Autodesk Fusion 360 part; units mm, degrees
(part 2 of 5)
  line L99 (217.2044, 94.7987, -0.5425) -> (214.1574, 88.9606, -0.5425)
  line L100 (229.1883, 17.794, -0.5425) -> (214.0829, 45.1294, -0.5425)
  line L101 (210.1198, 46.3093, -0.5425) -> (201.6545, 41.8242, -0.5425)
  line L102 (293.4635, 57.0179, -0.5425) -> (293.4635, 72.1916, -0.5425)
  arc A98 through (216.7158, 52.5703, -0.5425) (214.8476, 50.3729, -0.5425) (215.1327, 47.5028, -0.5425)
  arc A99 through (214.1574, 88.9606, -0.5425) (214.0147, 86.5484, -0.5425) (215.7224, 84.8389, -0.5425)
  line L103 (226.5548, 84.1235, -0.5425) -> (230.7717, 91.8438, -0.5425)
  line L104 (201.0039, 43.5591, -0.5425) -> (211.2158, 49.0246, -0.5425)
  line L105 (199.3291, 37.4177, -0.5425) -> (201.7431, 16.0362, -0.5425)
  line L106 (208.6237, 83.9074, -0.5425) -> (198.0965, 82.5311, -0.5425)
  line L107 (231.3102, 98.4094, -0.5425) -> (230.7073, 100.1344, -0.5425)
  line L108 (222.0557, 80.2922, -0.5425) -> (213.4569, 83.3852, -0.5425)
  arc A100 through (296.5336, 106.6129, -0.5425) (295.8856, 108.1774, -0.5425) (294.3211, 108.8254, -0.5425)
  line L109 (215.1327, 47.5028, -0.5425) -> (232.5299, 15.7176, -0.5425)
  arc A101 through (273.8579, 106.3021, -0.5425) (270.4819, 104.7377, -0.5425) (269.4929, 101.1507, -0.5425)
  line L110 (235.2375, 65.7635, -0.5425) -> (228.2248, 77.4788, -0.5425)
  arc A102 through (211.2158, 49.0246, -0.5425) (213.0904, 51.5465, -0.5425) (212.3403, 54.5979, -0.5425)
  arc A103 through (292.1232, 53.2736, -0.5425) (293.1183, 55.0294, -0.5425) (293.4635, 57.0179, -0.5425)
  arc A104 through (196.4178, 13.4172, -0.5425) (198.5944, 14.376, -0.5425) (199.3562, 16.6291, -0.5425)
  arc A105 through (233.851, 97.2274, -0.5425) (234.7613, 95.834, -0.5425) (236.1917, 94.9829, -0.5425)
  line L111 (268.8676, 90.1351, -0.5425) -> (266.9865, 102.5405, -0.5425)
  line L112 (232.4628, 66.2602, -0.5425) -> (226.309, 76.7604, -0.5425)
  line L113 (274.4552, 82.2574, -0.5425) -> (287.9958, 78.9742, -0.5425)
  arc A106 through (235.8049, 106.3021, -0.5425) (232.7822, 104.7266, -0.5425) (232.3424, 101.3464, -0.5425)
  arc A107 through (231.2263, 62.1248, -0.5425) (232.744, 63.9235, -0.5425) (232.4628, 66.2602, -0.5425)
  arc A108 through (215.5, 95.6328, -0.5425) (215.8168, 97.3721, -0.5425) (215.0822, 98.9802, -0.5425)
  line L114 (211.2519, 87.5615, -0.5425) -> (215.5, 95.6328, -0.5425)
  arc A109 through (222.0059, 82.4452, -0.5425) (224.595, 82.4316, -0.5425) (226.5548, 84.1235, -0.5425)
  arc A110 through (209.3714, 105.3255, -0.5425) (208.3789, 106.0469, -0.5425) (207.1787, 106.3021, -0.5425)
  line L115 (232.339, 60.3964, -0.5425) -> (216.7158, 52.5703, -0.5425)
  line L116 (215.7224, 84.8389, -0.5425) -> (222.0059, 82.4452, -0.5425)
  arc A111 through (209.0833, 86.0187, -0.5425) (210.3515, 86.5316, -0.5425) (211.2519, 87.5615, -0.5425)
  arc A112 through (201.7431, 16.0362, -0.5425) (202.7091, 14.1673, -0.5425) (204.6745, 13.4172, -0.5425)
  spline S0 degree 5 poles (37.6621, 101.8013, -0.5425) (37.9412, 101.8066, -0.5298) (38.4481, 101.843, -0.5085) (39.0545, 101.9753, -0.4883) (39.5781, 102.2952, -0.4831) (39.8825, 102.8688, -0.5029) (39.9929, 103.5346, -0.5365) (40.0648, 104.211, -0.5713) (40.2254, 104.8318, -0.5972) (40.5423, 105.3622, -0.609) (41.0432, 105.7885, -0.6044) (41.5947, 106.045, -0.5876) (42.0909, 106.1912, -0.5678) (42.4578, 106.2685, -0.5514) (42.6502, 106.3021, -0.5425) knots 0 0 0 0 0 0 0.1 0.2 0.3 0.4 0.5 0.6 0.7 0.8 0.9 1 1 1 1 1 1
  line L117 (36.4174, 101.7778, -0.5988) -> (38.9069, 101.8248, -0.4861)
  line L118 (65.0016, 71.3547, -0.5425) -> (79.0443, 79.8182, -0.5425)
  point P0 (207.0175, 69.7948)
  point P1 (207.0175, 69.7948)
  point P2 (40.091, 104.2207)
ref_plane "WorkPlane3" through (-60.7921, 150, 14.512) normal (0.12473, 0, 0.992191) x (0, 1, 0)
sketch "Sketch13" plane through (0.8502, 0, 6.7629) normal (0.12473, 0, 0.992191) x (0, 1, 0)
  arc A0 through (128.5492, 107.9276, -0.5425) (126.6265, 107.2149, -0.5425) (125.6327, 105.4212, -0.5425)
  arc A1 through (146.4088, 56.3524, -0.5425) (149.6864, 55.4797, -0.5425) (152.619, 57.1839, -0.5425)
  arc A2 through (13.5344, 103.4268, -0.5425) (11.1356, 102.4332, -0.5425) (10.1419, 100.0343, -0.5425)
  line L0 (10.1419, 65.1989, -0.5425) -> (10.1419, 18.7302, -0.5425)
  arc A3 through (13.9723, 85.5184, -0.5425) (11.3447, 85.0798, -0.5425) (10.1419, 82.7029, -0.5425)
  arc A4 through (156.4587, 58.9806, -0.5425) (155.942, 56.5284, -0.5425) (157.4975, 54.5636, -0.5425)
  line L1 (294.3211, 12.6445, -0.5425) -> (9.3501, 12.6445, -0.5425)
  line L2 (10.1419, 100.0343, -0.5425) -> (10.1419, 91.4948, -0.5425)
  arc A5 through (123.35, 103.697, -0.5425) (122.4956, 106.6479, -0.5425) (119.7027, 107.9276, -0.5425)
  arc A6 through (10.1419, 18.7302, -0.5425) (11.222, 16.1227, -0.5425) (13.8294, 15.0427, -0.5425)
  arc A7 through (103.6411, 44.2546, -0.5425) (106.2902, 44.6336, -0.5425) (107.543, 46.9984, -0.5425)
  arc A8 through (116.5331, 76.1094, -0.5425) (112.392, 76.5395, -0.5425) (110.1305, 73.0437, -0.5425)
  arc A9 through (9.3501, 110.4509, -0.5425) (7.7856, 109.8029, -0.5425) (7.1376, 108.2384, -0.5425)
  line L3 (120.1949, 82.505, -0.5425) -> (123.35, 103.697, -0.5425)
  line L4 (125.6327, 105.4212, -0.5425) -> (121.5744, 78.7404, -0.5425)
  line L5 (10.9643, 77.8757, -0.5425) -> (50.5643, 16.3952, -0.5425)
  line L6 (108.7653, 39.733, -0.5425) -> (125.8648, 19.9201, -0.5425)
  line L7 (110.1305, 73.0437, -0.5425) -> (109.448, 44.8203, -0.5425)
  arc A10 through (115.2719, 78.7654, -0.5425) (118.4948, 79.6329, -0.5425) (120.1949, 82.505, -0.5425)
  line L8 (12.6248, 88.1163, -0.5425) -> (62.0516, 72.6514, -0.5425)
  line L9 (45.4146, 20.7352, -0.5425) -> (15.5677, 66.8029, -0.5425)
  line L10 (9.3501, 14.8498) -> (294.6499, 14.8498)
  line L11 (9.3501, 110.4509, -0.5425) -> (294.3211, 110.4509, -0.5425)
  arc A11 through (107.9965, 74.659, -0.5425) (107.159, 76.9469, -0.5425) (105.004, 78.0835, -0.5425)
  arc A12 through (121.5744, 78.7404, -0.5425) (121.89, 76.034, -0.5425) (123.5394, 73.8653, -0.5425)
  arc A13 through (15.5677, 66.8029, -0.5425) (12.2556, 68.0278, -0.5425) (10.1419, 65.1989, -0.5425)
  arc A14 through (127.0398, 21.5138, -0.5425) (129.4645, 20.4975, -0.5425) (131.7372, 21.8193, -0.5425)
  arc A15 through (109.448, 44.8203, -0.5425) (109.8778, 42.1553, -0.5425) (111.2377, 39.8234, -0.5425)
  line L12 (153.5813, 51.294, -0.5425) -> (133.0891, 19.5942, -0.5425)
  line L13 (61.4337, 70.6789, -0.5425) -> (13.9723, 85.5184, -0.5425)
  arc A16 through (108.7653, 39.733, -0.5425) (107.7529, 40.6338, -0.5425) (106.5409, 41.2402, -0.5425)
  line L14 (123.5394, 73.8653, -0.5425) -> (146.4088, 56.3524, -0.5425)
  line L15 (13.8294, 15.0427, -0.5425) -> (42.3199, 15.0427, -0.5425)
  line L16 (111.2377, 39.8234, -0.5425) -> (127.0398, 21.5138, -0.5425)
  line L17 (37.6621, 103.4268, -0.5425) -> (13.5344, 103.4268, -0.5425)
  arc A17 (7.1376, 17.0623) -> (9.3501, 14.8498) centre (9.3501, 17.0623) ccw
  arc A18 through (70.492, 52.7161, -0.5425) (70.5116, 54.0318, -0.5425) (70.1435, 55.2951, -0.5425)
  line L18 (131.7372, 21.8193, -0.5425) -> (148.5132, 47.3064, -0.5425)
  line L19 (172.3385, 107.9276, -0.5425) -> (128.5492, 107.9276, -0.5425)
  line L20 (156.4587, 58.9806, -0.5425) -> (176.5219, 85.5722, -0.5425)
  line L21 (296.8624, 17.0623) -> (296.8624, 110.4437)
  arc A19 through (180.1276, 15.0427, -0.5425) (182.5336, 16.2858, -0.5425) (182.9119, 18.9675, -0.5425)
  line L22 (236.4115, 15.0427, -0.5425) -> (249.3606, 15.0427, -0.5425)
  arc A20 through (214.0829, 46.7549, -0.5425) (212.3427, 48.1555, -0.5425) (210.1198, 47.9348, -0.5425)
  line L23 (236.9767, 94.2988, -0.5425) -> (263.2633, 85.8479, -0.5425)
  arc A21 through (239.2829, 63.0131, -0.5425) (235.7303, 63.0824, -0.5425) (232.339, 62.0219, -0.5425)
  arc A22 through (235.2375, 67.389, -0.5425) (236.4809, 66.0477, -0.5425) (238.1606, 65.3238, -0.5425)
  line L24 (201.0039, 45.1846, -0.5425) -> (211.2158, 50.6501, -0.5425)
  line L25 (204.6745, 15.0427, -0.5425) -> (226.6063, 15.0427, -0.5425)
  line L26 (191.3482, 44.4035, -0.5425) -> (178.6355, 45.2846, -0.5425)
  line L27 (262.6115, 107.9276, -0.5425) -> (235.8049, 107.9276, -0.5425)
  line L28 (249.4163, 63.057, -0.5425) -> (238.1606, 65.3238, -0.5425)
  arc A23 through (196.4178, 15.0427, -0.5425) (198.5944, 16.0015, -0.5425) (199.3562, 18.2546, -0.5425)
  line L29 (236.1917, 96.6084, -0.5425) -> (264.0999, 87.6951, -0.5425)
  arc A24 through (175.2679, 40.8003, -0.5425) (173.7034, 43.4764, -0.5425) (171.2495, 45.3704, -0.5425)
  line L30 (248.8594, 61.2625, -0.5425) -> (239.2829, 63.0131, -0.5425)
  arc A25 through (213.8317, 57.7017, -0.5425) (215.4931, 56.6815, -0.5425) (217.428, 56.9204, -0.5425)
  line L31 (210.1198, 47.9348, -0.5425) -> (201.6545, 43.4497, -0.5425)
  line L32 (256.3019, 30.8271, -0.5425) -> (252.4432, 57.5422, -0.5425)
  line L33 (229.1883, 19.4195, -0.5425) -> (214.0829, 46.7549, -0.5425)
  line L34 (190.7528, 73.975, -0.5425) -> (196.7325, 47.1438, -0.5425)
  line L35 (254.2531, 57.8338, -0.5425) -> (258.1218, 32.1079, -0.5425)
  line L36 (196.1913, 79.369, -0.5425) -> (213.8317, 57.7017, -0.5425)
  line L37 (212.3403, 56.2234, -0.5425) -> (195.9237, 76.4744, -0.5425)
  line L38 (275.8299, 35.0581, -0.5425) -> (292.1232, 54.8991, -0.5425)
  line L39 (296.5336, 108.2384, -0.5425) -> (296.5336, 14.857, -0.5425)
  line L40 (300.5325, 116.9713, -0.5425) -> (300.5325, 7.1103, -0.5425)
  line L41 (261.9665, 29.7462, -0.5425) -> (273.8014, 33.6658, -0.5425)
  arc A26 through (294.3211, 12.6445, -0.5425) (295.8856, 13.2925, -0.5425) (296.5336, 14.857, -0.5425)
  line L42 (274.4552, 83.8829, -0.5425) -> (287.9958, 80.5997, -0.5425)
  line L43 (289.9863, 78.1394, -0.5425) -> (277.0376, 80.9788, -0.5425)
  arc A27 through (293.4635, 47.0663, -0.5425) (291.9967, 49.1493, -0.5425) (289.5412, 48.4704, -0.5425)
  arc A28 through (290.5135, 15.0427, -0.5425) (292.5995, 15.9067, -0.5425) (293.4635, 17.9927, -0.5425)
  arc A29 through (176.2747, 88.2323, -0.5425) (177.0332, 89.7841, -0.5425) (177.1399, 91.508, -0.5425)
  line L44 (289.0385, 107.9276, -0.5425) -> (273.8579, 107.9276, -0.5425)
  line L45 (187.1226, 81.2581, -0.5425) -> (194.4335, 47.9794, -0.5425)
  arc A30 through (175.2618, 105.3735, -0.5425) (174.2794, 107.1991, -0.5425) (172.3385, 107.9276, -0.5425)
  line L46 (232.4628, 67.8857, -0.5425) -> (226.309, 78.3859, -0.5425)
  arc A31 through (180.3167, 107.9276, -0.5425) (178.0915, 106.9144, -0.5425) (177.3948, 104.5708, -0.5425)
  line L47 (255.7129, 18.0094, -0.5425) -> (257.7618, 23.6594, -0.5425)
  arc A32 through (79.0291, 81.4345, -0.5425) (80.4163, 82.7098, -0.5425) (81.1941, 84.4262, -0.5425)
  arc A33 through (85.3097, 80.4194, -0.5425) (82.1977, 80.2707, -0.5425) (79.3035, 79.1172, -0.5425)
  arc A34 through (67.2556, 20.1909, -0.5425) (68.2461, 16.6058, -0.5425) (71.6211, 15.0427, -0.5425)
  arc A35 through (64.1302, 68.3113, -0.5425) (63.0327, 69.7807, -0.5425) (61.4337, 70.6789, -0.5425)
  arc A36 (294.6499, 14.8498) -> (296.8624, 17.0623) centre (294.6499, 17.0623) ccw
  line L48 (77.6309, 51.2153, -0.5425) -> (106.5409, 41.2402, -0.5425)
  line L49 (85.3097, 80.4194, -0.5425) -> (105.004, 78.0835, -0.5425)
  line L50 (119.7027, 107.9276, -0.5425) -> (92.2179, 107.9276, -0.5425)
  line L51 (103.6411, 44.2546, -0.5425) -> (75.7593, 53.7636, -0.5425)
  line L52 (87.1104, 82.2687, -0.5425) -> (115.2719, 78.7654, -0.5425)
  line L53 (123.6315, 15.0427, -0.5425) -> (71.6211, 15.0427, -0.5425)
  arc A37 through (157.3818, 52.3291, -0.5425) (155.2835, 52.5387, -0.5425) (153.5813, 51.294, -0.5425)
  line L54 (3.4675, 116.9713, -0.5425) -> (300.5325, 116.9713, -0.5425)
  arc A38 through (216.7158, 54.1958, -0.5425) (214.8476, 51.9984, -0.5425) (215.1327, 49.1283, -0.5425)
  arc A39 through (196.7325, 47.1438, -0.5425) (198.3819, 45.1041, -0.5425) (201.0039, 45.1846, -0.5425)
  line L55 (173.0748, 46.7985, -0.5425) -> (157.4975, 54.5636, -0.5425)
  arc A40 through (181.0984, 42.9156, -0.5425) (178.5412, 41.7629, -0.5425) (178.1042, 38.9921, -0.5425)
  arc A41 through (173.0748, 46.7985, -0.5425) (175.7805, 45.7673, -0.5425) (178.6355, 45.2846, -0.5425)
  line L56 (135.5665, 15.0427, -0.5425) -> (180.1276, 15.0427, -0.5425)
  line L57 (178.1042, 38.9921, -0.5425) -> (185.8555, 17.0116, -0.5425)
  line L58 (217.428, 56.9204, -0.5425) -> (231.2263, 63.7503, -0.5425)
  line L59 (232.339, 62.0219, -0.5425) -> (216.7158, 54.1958, -0.5425)
  arc A42 through (201.6545, 43.4497, -0.5425) (199.8127, 41.6049, -0.5425) (199.3291, 39.0432, -0.5425)
  arc A43 through (61.1239, 15.0427, -0.5425) (63.5088, 15.9177, -0.5425) (64.7618, 18.1275, -0.5425)
  arc A44 through (50.5643, 16.3952, -0.5425) (51.6319, 15.4028, -0.5425) (53.0443, 15.0427, -0.5425)
  arc A45 through (77.6309, 51.2153, -0.5425) (73.9232, 50.8341, -0.5425) (71.8221, 47.7555, -0.5425)
  line L60 (64.7618, 18.1275, -0.5425) -> (70.492, 52.7161, -0.5425)
  line L61 (53.0443, 15.0427, -0.5425) -> (61.1239, 15.0427, -0.5425)
  line L62 (88.0477, 104.6024, -0.5425) -> (83.9707, 86.7489, -0.5425)
  line L63 (71.4916, 57.5515, -0.5425) -> (66.9703, 66.9675, -0.5425)
  line L64 (81.7514, 107.9276, -0.5425) -> (42.6502, 107.9276, -0.5425)
  arc A46 through (68.665, 72.6667, -0.5425) (66.7178, 70.1441, -0.5425) (66.9703, 66.9675, -0.5425)
  arc A47 through (71.4916, 57.5515, -0.5425) (73.2442, 55.228, -0.5425) (75.7593, 53.7636, -0.5425)
  arc A48 through (232.5299, 17.3431, -0.5425) (234.1555, 15.661, -0.5425) (236.4115, 15.0427, -0.5425)
  arc A49 through (201.7431, 17.6617, -0.5425) (202.7091, 15.7928, -0.5425) (204.6745, 15.0427, -0.5425)
  arc A50 through (231.2263, 63.7503, -0.5425) (232.744, 65.549, -0.5425) (232.4628, 67.8857, -0.5425)
  line L65 (199.3291, 39.0432, -0.5425) -> (201.7431, 17.6617, -0.5425)
  line L66 (199.3562, 18.2546, -0.5425) -> (197.4845, 39.2503, -0.5425)
  arc A51 through (211.2158, 50.6501, -0.5425) (213.0904, 53.172, -0.5425) (212.3403, 56.2234, -0.5425)
  line L67 (171.2495, 45.3704, -0.5425) -> (157.3818, 52.3291, -0.5425)
  line L68 (7.1376, 110.4437) -> (7.1376, 17.0623)
  arc A52 through (62.0516, 72.6514, -0.5425) (63.5927, 72.5096, -0.5425) (65.0563, 73.0125, -0.5425)
  arc A53 through (42.3199, 15.0427, -0.5425) (45.5596, 16.9689, -0.5425) (45.4146, 20.7352, -0.5425)
  line L69 (81.1941, 84.4262, -0.5425) -> (85.4902, 103.2388, -0.5425)
  line L70 (68.665, 72.6667, -0.5425) -> (79.3035, 79.1172, -0.5425)
  arc A54 through (83.9707, 86.7489, -0.5425) (84.5459, 83.8117, -0.5425) (87.1104, 82.2687, -0.5425)
  line L71 (67.2556, 20.1909, -0.5425) -> (71.8221, 47.7555, -0.5425)
  line L72 (65.0016, 72.9802, -0.5425) -> (79.0443, 81.4437, -0.5425)
  line L73 (70.1435, 55.2951, -0.5425) -> (64.1302, 68.3113, -0.5425)
  arc A55 through (85.4902, 103.2388, -0.5425) (84.7499, 106.4835, -0.5425) (81.7514, 107.9276, -0.5425)
  arc A56 through (92.2179, 107.9276, -0.5425) (89.5511, 106.9945, -0.5425) (88.0477, 104.6024, -0.5425)
  arc A57 through (226.6063, 15.0427, -0.5425) (229.1471, 16.4937, -0.5425) (229.1883, 19.4195, -0.5425)
  arc A58 through (191.3482, 44.4035, -0.5425) (193.7858, 45.4194, -0.5425) (194.4335, 47.9794, -0.5425)
  arc A59 through (197.4845, 39.2503, -0.5425) (196.6144, 41.092, -0.5425) (194.7583, 41.9308, -0.5425)
  line L74 (215.1327, 49.1283, -0.5425) -> (232.5299, 17.3431, -0.5425)
  line L75 (194.7583, 41.9308, -0.5425) -> (181.0984, 42.9156, -0.5425)
  arc A60 through (185.8555, 17.0116, -0.5425) (186.9334, 15.5847, -0.5425) (188.6375, 15.0427, -0.5425)
  arc A61 through (133.0891, 19.5942, -0.5425) (132.9755, 16.5823, -0.5425) (135.5665, 15.0427, -0.5425)
  line L76 (276.3301, 32.1764, -0.5425) -> (290.2479, 30.3805, -0.5425)
  arc A62 through (276.3301, 32.1764, -0.5425) (275.6694, 32.187, -0.5425) (275.0229, 32.0503, -0.5425)
  line L77 (289.5412, 48.4704, -0.5425) -> (280.1951, 37.0893, -0.5425)
  arc A63 through (198.0965, 84.1566, -0.5425) (195.738, 82.3223, -0.5425) (196.1913, 79.369, -0.5425)
  arc A64 through (287.9958, 80.5997, -0.5425) (291.7741, 81.422, -0.5425) (293.4635, 84.9001, -0.5425)
  line L78 (261.9099, 27.6959, -0.5425) -> (275.0229, 32.0503, -0.5425)
  arc A65 through (293.4635, 26.7234, -0.5425) (292.5453, 29.1583, -0.5425) (290.2479, 30.3805, -0.5425)
  line L79 (180.9121, 89.4237, -0.5425) -> (188.1391, 86.2233, -0.5425)
  arc A66 through (265.809, 82.6487, -0.5425) (265.0201, 84.6334, -0.5425) (263.2633, 85.8479, -0.5425)
  line L80 (235.2375, 67.389, -0.5425) -> (228.2248, 79.1043, -0.5425)
  arc A67 through (280.1951, 37.0893, -0.5425) (279.848, 34.8702, -0.5425) (281.6207, 33.491, -0.5425)
  line L81 (182.035, 86.864, -0.5425) -> (183.2206, 86.2706, -0.5425)
  arc A68 through (290.9668, 32.2801, -0.5425) (292.7116, 32.8124, -0.5425) (293.4635, 34.4743, -0.5425)
  arc A69 through (255.7129, 18.0094, -0.5425) (255.9812, 15.9851, -0.5425) (257.7929, 15.0427, -0.5425)
  line L82 (253.5627, 18.0811, -0.5425) -> (255.7697, 24.7696, -0.5425)
  line L83 (208.6237, 85.5329, -0.5425) -> (198.0965, 84.1566, -0.5425)
  arc A70 through (209.3714, 106.951, -0.5425) (208.3789, 107.6724, -0.5425) (207.1787, 107.9276, -0.5425)
  arc A71 through (249.3606, 15.0427, -0.5425) (251.9533, 15.8818, -0.5425) (253.5627, 18.0811, -0.5425)
  line L84 (281.6207, 33.491, -0.5425) -> (290.9668, 32.2801, -0.5425)
  arc A72 through (292.1232, 54.8991, -0.5425) (293.1183, 56.6549, -0.5425) (293.4635, 58.6434, -0.5425)
  line L85 (293.4635, 34.4743, -0.5425) -> (293.4635, 47.0663, -0.5425)
  arc A73 through (255.7697, 24.7696, -0.5425) (256.3873, 27.7675, -0.5425) (256.3019, 30.8271, -0.5425)
  arc A74 through (258.1218, 32.1079, -0.5425) (259.4949, 30.033, -0.5425) (261.9665, 29.7462, -0.5425)
  line L86 (265.809, 82.6487, -0.5425) -> (265.9528, 80.9526, -0.5425)
  arc A75 through (273.8014, 33.6658, -0.5425) (274.9144, 34.2181, -0.5425) (275.8299, 35.0581, -0.5425)
  line L87 (264.5468, 76.607, -0.5425) -> (254.3494, 64.7515, -0.5425)
  arc A76 through (213.4569, 85.0107, -0.5425) (211.0714, 85.5603, -0.5425) (208.6237, 85.5329, -0.5425)
  arc A77 through (261.9099, 27.6959, -0.5425) (259.3727, 26.1536, -0.5425) (257.7618, 23.6594, -0.5425)
  line L88 (293.4635, 26.7234, -0.5425) -> (293.4635, 17.9927, -0.5425)
  arc A78 through (209.0833, 87.6442, -0.5425) (210.3515, 88.1571, -0.5425) (211.2519, 89.187, -0.5425)
  line L89 (290.5135, 15.0427, -0.5425) -> (257.7929, 15.0427, -0.5425)
  arc A79 through (249.4163, 63.057, -0.5425) (252.1126, 63.2354, -0.5425) (254.3494, 64.7515, -0.5425)
  line L90 (177.3948, 104.5708, -0.5425) -> (179.1848, 91.7143, -0.5425)
  line L91 (269.2803, 78.4929, -0.5425) -> (256.0736, 63.8745, -0.5425)
  arc A80 through (182.035, 86.864, -0.5425) (179.0447, 87.2154, -0.5425) (176.5219, 85.5722, -0.5425)
  arc A81 through (188.1391, 86.2233, -0.5425) (191.1487, 85.3739, -0.5425) (194.2757, 85.4006, -0.5425)
  line L92 (269.4929, 102.7762, -0.5425) -> (272.2404, 86.2656, -0.5425)
  line L93 (228.1101, 84.2056, -0.5425) -> (232.6022, 92.5381, -0.5425)
  arc A82 through (187.1226, 81.2581, -0.5425) (185.7389, 84.206, -0.5425) (183.2206, 86.2706, -0.5425)
  arc A83 through (179.1848, 91.7143, -0.5425) (179.7513, 90.3449, -0.5425) (180.9121, 89.4237, -0.5425)
  line L94 (207.1787, 107.9276, -0.5425) -> (180.3167, 107.9276, -0.5425)
  arc A84 through (220.6389, 100.0016, -0.5425) (218.6659, 98.4584, -0.5425) (217.2044, 96.4242, -0.5425)
  line L95 (194.2757, 85.4006, -0.5425) -> (209.0833, 87.6442, -0.5425)
  line L96 (177.1399, 91.508, -0.5425) -> (175.2618, 105.3735, -0.5425)
  line L97 (293.4635, 84.9001, -0.5425) -> (293.4635, 103.5026, -0.5425)
  arc A85 through (252.4432, 57.5422, -0.5425) (251.2505, 59.9796, -0.5425) (248.8594, 61.2625, -0.5425)
  arc A86 through (272.2404, 86.2656, -0.5425) (272.9897, 84.7413, -0.5425) (274.4552, 83.8829, -0.5425)
  arc A87 through (195.9237, 76.4744, -0.5425) (192.3483, 77.2728, -0.5425) (190.7528, 73.975, -0.5425)
  arc A88 through (236.9767, 94.2988, -0.5425) (234.4712, 94.2091, -0.5425) (232.6022, 92.5381, -0.5425)
  line L98 (226.5548, 85.749, -0.5425) -> (230.7717, 93.4693, -0.5425)
  line L99 (293.4635, 58.6434, -0.5425) -> (293.4635, 73.8171, -0.5425)
  line L100 (211.2519, 89.187, -0.5425) -> (215.5, 97.2583, -0.5425)
  line L101 (215.7224, 86.4644, -0.5425) -> (222.0059, 84.0707, -0.5425)
  arc A89 through (293.4635, 103.5026, -0.5425) (292.1675, 106.6315, -0.5425) (289.0385, 107.9276, -0.5425)
  arc A90 through (277.0376, 80.9788, -0.5425) (272.8243, 80.7801, -0.5425) (269.2803, 78.4929, -0.5425)
  arc A91 through (230.7073, 101.7599, -0.5425) (228.9517, 103.5512, -0.5425) (226.4521, 103.3439, -0.5425)
  arc A92 through (273.8579, 107.9276, -0.5425) (270.4819, 106.3632, -0.5425) (269.4929, 102.7762, -0.5425)
  arc A93 through (214.1574, 90.5861, -0.5425) (214.0147, 88.1739, -0.5425) (215.7224, 86.4644, -0.5425)
  arc A94 through (293.4635, 73.8171, -0.5425) (292.4863, 76.5907, -0.5425) (289.9863, 78.1394, -0.5425)
  arc A95 through (215.5, 97.2583, -0.5425) (215.8168, 98.9976, -0.5425) (215.0822, 100.6057, -0.5425)
  arc A96 through (296.5336, 108.2384, -0.5425) (295.8856, 109.8029, -0.5425) (294.3211, 110.4509, -0.5425)
  arc A97 through (222.0059, 84.0707, -0.5425) (224.595, 84.0571, -0.5425) (226.5548, 85.749, -0.5425)
  line L102 (232.3424, 102.9719, -0.5425) -> (233.851, 98.8529, -0.5425)
  line L103 (222.0557, 81.9177, -0.5425) -> (213.4569, 85.0107, -0.5425)
  arc A98 through (235.8049, 107.9276, -0.5425) (232.7822, 106.3521, -0.5425) (232.3424, 102.9719, -0.5425)
  line L104 (231.3102, 100.0349, -0.5425) -> (230.7073, 101.7599, -0.5425)
  arc A99 (296.8624, 110.4437) -> (294.6499, 112.6562) centre (294.6499, 110.4437) ccw
  arc A100 through (230.7717, 93.4693, -0.5425) (231.7374, 96.695, -0.5425) (231.3102, 100.0349, -0.5425)
  line L105 (217.2044, 96.4242, -0.5425) -> (214.1574, 90.5861, -0.5425)
  arc A101 through (226.309, 78.3859, -0.5425) (224.4925, 80.5253, -0.5425) (222.0557, 81.9177, -0.5425)
  line L106 (215.0822, 100.6057, -0.5425) -> (209.3714, 106.951, -0.5425)
  line L107 (268.8676, 91.7606, -0.5425) -> (266.9865, 104.166, -0.5425)
  arc A102 through (233.851, 98.8529, -0.5425) (234.7613, 97.4595, -0.5425) (236.1917, 96.6084, -0.5425)
  line L108 (226.4521, 103.3439, -0.5425) -> (220.6389, 100.0016, -0.5425)
  arc A103 through (256.0736, 63.8745, -0.5425) (254.4848, 61.0587, -0.5425) (254.2531, 57.8338, -0.5425)
  arc A104 through (264.5468, 76.607, -0.5425) (265.6874, 78.6383, -0.5425) (265.9528, 80.9526, -0.5425)
  arc A105 through (266.9865, 104.166, -0.5425) (265.4964, 106.8579, -0.5425) (262.6115, 107.9276, -0.5425)
  arc A106 through (264.0999, 87.6951, -0.5425) (267.6144, 88.4019, -0.5425) (268.8676, 91.7606, -0.5425)
  arc A107 through (228.1101, 84.2056, -0.5425) (227.4932, 81.6398, -0.5425) (228.2248, 79.1043, -0.5425)
  line L109 (182.9119, 18.9675, -0.5425) -> (175.2679, 40.8003, -0.5425)
  line L110 (188.6375, 15.0427, -0.5425) -> (196.4178, 15.0427, -0.5425)
  line L111 (152.619, 57.1839, -0.5425) -> (176.2747, 88.2323, -0.5425)
  line L112 (10.1419, 82.7029, -0.5425) -> (10.1419, 80.6712, -0.5425)
  line L113 (3.4675, 7.1103, -0.5425) -> (3.4675, 116.9713, -0.5425)
  arc A108 through (123.6315, 15.0427, -0.5425) (126.3137, 16.7645, -0.5425) (125.8648, 19.9201, -0.5425)
  arc A109 through (10.1419, 91.4948, -0.5425) (10.8294, 89.3984, -0.5425) (12.6248, 88.1163, -0.5425)
  line L114 (107.9965, 74.659, -0.5425) -> (107.543, 46.9984, -0.5425)
  arc A110 through (148.5132, 47.3064, -0.5425) (149.0689, 49.9488, -0.5425) (147.6751, 52.2615, -0.5425)
  arc A111 through (10.1419, 80.6712, -0.5425) (10.3518, 79.2143, -0.5425) (10.9643, 77.8757, -0.5425)
  line L115 (7.1376, 14.857, -0.5425) -> (7.1376, 108.2384, -0.5425)
  arc A112 through (7.1376, 14.857, -0.5425) (7.7856, 13.2925, -0.5425) (9.3501, 12.6445, -0.5425)
  line L116 (147.6751, 52.2615, -0.5425) -> (116.5331, 76.1094, -0.5425)
  line L117 (37.6527, 103.4268, -0.5425) -> (42.657, 107.9276, -0.5425)
  point P0 (207.0175, 71.4203)
  point P1 (207.0175, 71.4203)
extrude "Extrude4" cut sketch "Sketch13" against normal through all contours A0 A1 L4 A12 L14 L19 A29 A30 L96 L111 | A2 L2 L8 L17 A32 L64 A52 L69 L72 A55 A109 L117 | L0 A6 L9 A13 L15 A53 | A3 L5 L13 A18 A35 A43 A44 L60 L61 L73 L112 A111 | A4 L20 L26 L45 L55 A41 A58 L81 A80 A82 | A5 L3 A10 L50 L52 L62 A54 A56 | A7 A11 A33 L49 L51 L63 A46 A47 L70 L114 | A8 L7 A14 A15 L16 L18 A110 L116 | L6 A16 A34 L48 L53 A45 L71 A108 | L12 A19 A24 A37 L56 L67 A61 L109 | L22 A21 L30 L32 A38 L59 A48 L74 L82 A71 A73 A85 | A20 L25 L31 L33 A42 A49 L65 A57 | L23 A22 L28 A66 L80 L86 L87 A79 L93 A88 A104 A107 | L24 L34 L37 A39 A51 A87 | L27 L29 L102 A98 L107 A102 A105 A106 | A23 A40 L57 L66 A59 L75 A60 L110 | A25 L36 L46 L58 A50 A63 L83 A76 L103 A101 | L35 L38 L41 L43 A72 A74 A75 L91 L99 A90 A94 A103 | L42 L44 A64 L92 L97 A86 A89 A92 | A27 L77 A67 A68 L84 L85 | A28 L47 L76 A62 L78 A65 A69 A77 L88 L89 | A31 L79 A70 A78 L90 A81 A83 L94 L95 L100 A95 L106 | A84 L98 L101 A91 A93 A97 L104 A100 L105 L108 in plane through (0.7825, 0, 6.2246) normal (0.12473, 0, 0.992191)
sketch "Sketch14" plane through (0, 0, 0) normal (0, -1, 0) x (1, 0, 0)
  line L0 (-113.7873, 37.3) -> (-113.7873, 4.9975)
  line L1 (-113.7873, 4.9975) -> (-4.7873, 4.9975)
  line L2 (-4.7873, 4.9975) -> (-4.7873, 23.5975)
  line L3 (-4.7873, 23.5975) -> (-113.7873, 37.3)
sketch "Sketch15" plane through (0, 0, 0) normal (0, 0, 1) x (1, 0, 0)
  line L0 (5.3988, -2.1298) -> (5.3988, 1.5536)
  line L1 (5.3988, 1.5536) -> (6.4633, 1.4209)
  line L2 (6.4633, 1.4209) -> (6.0119, -2.2014)
  line L3 (6.0119, -2.2014) -> (5.3988, -2.1298)
  line L4 (5.4744, 1.348) -> (5.5749, 1.5095) construction
  line L5 (5.5749, 1.5095) -> (5.9354, 1.3104) construction
  line L6 (5.9354, 1.3104) -> (5.4453, 1.1367) construction
  line L7 (5.4453, 1.1367) -> (5.4378, 1.2494) construction
  line L8 (5.4378, 1.2494) -> (5.4744, 1.348) construction
  spline S0 degree 5 poles (5.4744, 1.348) (5.5749, 1.5095) (5.9354, 1.3104) (5.4453, 1.1367) (5.4378, 1.2494) (5.4744, 1.348) knots 0 0 0 0 0 0 1 1 1 1 1 1
  line L9 (6.0311, 1.103) -> (6.0048, 1.3059) construction
  line L10 (6.0048, 1.3059) -> (6.0442, 1.46) construction
  line L11 (6.0442, 1.46) -> (5.4771, 1.1925) construction
  line L12 (5.4771, 1.1925) -> (5.3709, 1.0098) construction
  line L13 (5.3709, 1.0098) -> (5.5225, 0.9394) construction
  line L14 (5.5225, 0.9394) -> (5.6861, 0.8534) construction
  line L15 (5.6861, 0.8534) -> (6.0526, 0.9979) construction
  line L16 (6.0526, 0.9979) -> (6.0311, 1.103) construction
  spline S1 degree 5 poles (6.0311, 1.103) (6.0048, 1.3059) (6.0442, 1.46) (5.4771, 1.1925) (5.3709, 1.0098) (5.5225, 0.9394) (5.6861, 0.8534) (6.0526, 0.9979) (6.0311, 1.103) knots 0 0 0 0 0 0 0.25 0.5 0.75 1 1 1 1 1 1
  line L17 (6.1058, 0.8886) -> (6.162, 0.6486)
  line L18 (6.2944, 0.6369) -> (6.2967, 0.642)
  line L19 (6.3105, 0.694) -> (6.3258, 0.826)
  line L20 (6.2336, 0.9612) -> (6.1918, 0.9722)
  arc A0 (6.1918, 0.9722) -> (6.1058, 0.8886) centre (6.1739, 0.9046) ccw
  arc A1 (6.162, 0.6486) -> (6.2944, 0.6369) centre (6.2301, 0.6646) ccw
  arc A2 (6.2967, 0.642) -> (6.3105, 0.694) centre (6.1268, 0.7153) ccw
  arc A3 (6.3258, 0.826) -> (6.2336, 0.9612) centre (6.2016, 0.8403) ccw
  line L21 (5.9923, 0.0338) -> (6.0698, -0.2718)
  line L22 (6.1873, -0.266) -> (6.2399, 0.0832)
  line L23 (6.2112, 0.22) -> (6.1931, 0.2485)
  line L24 (6.0168, 0.2345) -> (6.0062, 0.21)
  arc A4 (6.1931, 0.2485) -> (6.0168, 0.2345) centre (6.1086, 0.195) ccw
  arc A5 (6.0062, 0.21) -> (5.9923, 0.0338) centre (6.2588, 0.1014) ccw
  arc A6 (6.2399, 0.0832) -> (6.2112, 0.22) centre (6.0422, 0.1131) ccw
  arc A7 (6.0698, -0.2718) -> (6.1873, -0.266) centre (6.1279, -0.257) ccw
  line L25 (5.9776, -1.9957) -> (6.0438, -1.4551)
  line L26 (5.933, -1.3436) -> (5.8966, -1.3479)
  line L27 (5.6749, -1.4635) -> (5.5171, -1.6418)
  line L28 (5.4543, -1.8075) -> (5.4543, -1.9385)
  line L29 (5.5405, -2.0375) -> (5.8646, -2.0826)
  arc A8 (6.0438, -1.4551) -> (5.933, -1.3436) centre (5.9445, -1.443) ccw
  arc A9 (5.8966, -1.3479) -> (5.6749, -1.4635) centre (5.937, -1.6955) ccw
  arc A10 (5.5171, -1.6418) -> (5.4543, -1.8075) centre (5.7043, -1.8075) ccw
  arc A11 (5.8646, -2.0826) -> (5.9776, -1.9957) centre (5.8784, -1.9835) ccw
  arc A12 (5.4543, -1.9385) -> (5.5405, -2.0375) centre (5.5543, -1.9385) ccw
  line L30 (5.716, -0.8769) -> (5.7261, -1.2218)
  line L31 (5.6538, -1.4051) -> (5.5473, -1.5125)
  line L32 (5.4703, -1.4808) -> (5.4703, -0.8771)
  line L33 (5.5453, -0.7803) -> (5.5472, -0.7798)
  line L34 (5.5472, -0.7798) -> (5.6172, -0.7798)
  line L35 (5.6172, -0.7798) -> (5.6161, -0.7798)
  arc A13 (5.5453, -0.7803) -> (5.4703, -0.8771) centre (5.5703, -0.8771) ccw
  arc A14 (5.716, -0.8769) -> (5.6161, -0.7798) centre (5.6161, -0.8798) ccw
  arc A15 (5.6538, -1.4051) -> (5.7261, -1.2218) centre (5.4762, -1.2291) ccw
  arc A16 (5.4703, -1.4808) -> (5.5473, -1.5125) centre (5.5153, -1.4808) ccw
  line L36 (5.7779, -0.6031) -> (5.7773, -1.1532)
  line L37 (5.9091, -1.2844) -> (6.0011, -1.2758)
  line L38 (6.0011, -1.2758) -> (5.978, -1.278)
  line L39 (6.0677, -1.1924) -> (6.1601, -0.5408)
  line L40 (6.0692, -0.4571) -> (5.8557, -0.5057)
  arc A17 (5.7773, -1.1532) -> (5.8256, -1.2636) centre (5.9273, -1.1534) ccw
  arc A18 (5.8256, -1.2636) -> (5.9091, -1.2844) centre (5.897, -1.155) ccw
  arc A19 (5.8557, -0.5057) -> (5.7779, -0.6031) centre (5.8779, -0.6032) ccw
  arc A20 (5.978, -1.278) -> (6.0677, -1.1924) centre (5.9686, -1.1784) ccw
  arc A21 (6.1601, -0.5408) -> (6.0692, -0.4571) centre (6.0858, -0.5303) ccw
  line L41 (5.4668, -0.5654) -> (5.5025, -0.4813) construction
  line L42 (5.5025, -0.4813) -> (5.6981, -0.5066) construction
  line L43 (5.6981, -0.5066) -> (5.7507, -0.5528) construction
  line L44 (5.7507, -0.5528) -> (5.839, -0.8009) construction
  line L45 (5.839, -0.8009) -> (5.4416, -0.7358) construction
  line L46 (5.4416, -0.7358) -> (5.4668, -0.5654) construction
  spline S2 degree 5 poles (5.4668, -0.5654) (5.5025, -0.4813) (5.6981, -0.5066) (5.7507, -0.5528) (5.839, -0.8009) (5.4416, -0.7358) (5.4668, -0.5654) knots 0 0 0 0 0 0 0.5 1 1 1 1 1 1
  line L47 (5.4584, 0.0475) -> (5.4584, -0.329)
  line L48 (5.5834, -0.454) -> (5.6398, -0.454)
  line L49 (5.8754, -0.4279) -> (5.9471, -0.4118)
  line L50 (6.0217, -0.2878) -> (5.9448, -0.0066)
  line L51 (5.8693, 0.1148) -> (5.7172, 0.2492)
  line L52 (5.5703, 0.2333) -> (5.4776, 0.1064)
  arc A22 (5.4776, 0.1064) -> (5.4584, 0.0475) centre (5.5584, 0.0475) ccw
  arc A23 (5.7172, 0.2492) -> (5.5703, 0.2333) centre (5.651, 0.1743) ccw
  arc A24 (5.9448, -0.0066) -> (5.8693, 0.1148) centre (5.7037, -0.0725) ccw
  arc A25 (5.9471, -0.4118) -> (6.0217, -0.2878) centre (5.9252, -0.3142) ccw
  arc A26 (5.6398, -0.454) -> (5.8754, -0.4279) centre (5.6398, 0.621) ccw
  arc A27 (5.4584, -0.329) -> (5.5834, -0.454) centre (5.5834, -0.329) ccw
  line L53 (5.4649, 0.3902) -> (5.4649, 0.2831) construction
  line L54 (5.4649, 0.2831) -> (5.471, 0.2306) construction
  line L55 (5.471, 0.2306) -> (5.5942, 0.2286) construction
  line L56 (5.5942, 0.2286) -> (5.6366, 0.3538) construction
  line L57 (5.6366, 0.3538) -> (5.5518, 0.467) construction
  line L58 (5.5518, 0.467) -> (5.4649, 0.3902) construction
  spline S3 degree 5 poles (5.4649, 0.3902) (5.4649, 0.2831) (5.471, 0.2306) (5.5942, 0.2286) (5.6366, 0.3538) (5.5518, 0.467) (5.4649, 0.3902) knots 0 0 0 0 0 0 0.5 1 1 1 1 1 1
  line L59 (6.0183, 0.4104) -> (6.0284, 0.4589) construction
  line L60 (6.0284, 0.4589) -> (6.0769, 0.5134) construction
  line L61 (6.0769, 0.5134) -> (6.1557, 0.5033) construction
  line L62 (6.1557, 0.5033) -> (6.2001, 0.4286) construction
  line L63 (6.2001, 0.4286) -> (6.1436, 0.3458) construction
  line L64 (6.1436, 0.3458) -> (6.0345, 0.3498) construction
  line L65 (6.0345, 0.3498) -> (6.0183, 0.4104) construction
  spline S4 degree 5 poles (6.0183, 0.4104) (6.0284, 0.4589) (6.0769, 0.5134) (6.1557, 0.5033) (6.2001, 0.4286) (6.1436, 0.3458) (6.0345, 0.3498) (6.0183, 0.4104) knots 0 0 0 0 0 0 0.333333 0.666667 1 1 1 1 1 1
  line L66 (5.8042, 0.2629) -> (5.883, 0.1599) construction
  line L67 (5.883, 0.1599) -> (5.9598, 0.164) construction
  line L68 (5.9598, 0.164) -> (5.9961, 0.2932) construction
  line L69 (5.9961, 0.2932) -> (5.9699, 0.4245) construction
  line L70 (5.9699, 0.4245) -> (5.8406, 0.5659) construction
  line L71 (5.8406, 0.5659) -> (5.7517, 0.4972) construction
  line L72 (5.7517, 0.4972) -> (5.7133, 0.4003) construction
  line L73 (5.7133, 0.4003) -> (5.7214, 0.3114) construction
  line L74 (5.7214, 0.3114) -> (5.8042, 0.2629) construction
  spline S5 degree 5 poles (5.8042, 0.2629) (5.883, 0.1599) (5.9598, 0.164) (5.9961, 0.2932) (5.9699, 0.4245) (5.8406, 0.5659) (5.7517, 0.4972) (5.7133, 0.4003) (5.7214, 0.3114) (5.8042, 0.2629) knots 0 0 0 0 0 0 0.2 0.4 0.6 0.8 1 1 1 1 1 1
  line L75 (5.9436, 0.9174) -> (6.0587, 0.9154) construction
  line L76 (6.0587, 0.9154) -> (6.089, 0.7639) construction
  line L77 (6.089, 0.7639) -> (6.1436, 0.5518) construction
  line L78 (6.1436, 0.5518) -> (6.0103, 0.5215) construction
  line L79 (6.0103, 0.5215) -> (5.8911, 0.5356) construction
  line L80 (5.8911, 0.5356) -> (5.8426, 0.6083) construction
  line L81 (5.8426, 0.6083) -> (5.8042, 0.7215) construction
  line L82 (5.8042, 0.7215) -> (5.8426, 0.8527) construction
  line L83 (5.8426, 0.8527) -> (5.9436, 0.9174) construction
  spline S6 degree 5 poles (5.9436, 0.9174) (6.0587, 0.9154) (6.089, 0.7639) (6.1436, 0.5518) (6.0103, 0.5215) (5.8911, 0.5356) (5.8426, 0.6083) (5.8042, 0.7215) (5.8426, 0.8527) (5.9436, 0.9174) knots 0 0 0 0 0 0 0.2 0.4 0.6 0.8 1 1 1 1 1 1
  line L84 (5.472, 0.7736) -> (5.465, 0.5843)
  line L85 (5.5042, 0.4886) -> (5.512, 0.4812)
  line L86 (5.6401, 0.4546) -> (5.6373, 0.4536)
  line L87 (5.7362, 0.5433) -> (5.7412, 0.554)
  line L88 (5.7565, 0.7493) -> (5.7539, 0.7579)
  line L89 (5.6738, 0.8412) -> (5.6038, 0.8647)
  arc A28 (5.6038, 0.8647) -> (5.472, 0.7736) centre (5.572, 0.7699) ccw
  arc A29 (5.465, 0.5843) -> (5.5042, 0.4886) centre (5.5899, 0.5796) ccw
  arc A30 (5.512, 0.4812) -> (5.6401, 0.4546) centre (5.5978, 0.5722) ccw
  arc A31 (5.6373, 0.4536) -> (5.7362, 0.5433) centre (5.578, 0.6182) ccw
  arc A32 (5.7412, 0.554) -> (5.7565, 0.7493) centre (5.4927, 0.6717) ccw
  arc A33 (5.7539, 0.7579) -> (5.6738, 0.8412) centre (5.634, 0.7227) ccw
  line L90 (6.0842, 1.2372) -> (6.0915, 1.1979)
  line L91 (6.2705, 1.0353) -> (6.2729, 1.0351)
  line L92 (6.3542, 1.1032) -> (6.3628, 1.2003)
  line L93 (6.2787, 1.3079) -> (6.1696, 1.325)
  arc A34 (6.1696, 1.325) -> (6.0842, 1.2372) centre (6.158, 1.2509) ccw
  arc A35 (6.3628, 1.2003) -> (6.2787, 1.3079) centre (6.2632, 1.2091) ccw
  arc A36 (6.2729, 1.0351) -> (6.3542, 1.1032) centre (6.2795, 1.1098) ccw
  arc A37 (6.0915, 1.1979) -> (6.2705, 1.0353) centre (6.2882, 1.2345) ccw
  line L94 (5.9709, 1.4823) -> (5.519, -2.1438)
  dimension "d348" = 0.07
  dimension "d349" = 0.07
  dimension "d350" = 0.185
  dimension "d351" = 0.125
  dimension "d352" = 0.1
  dimension "d353" = 0.275
  dimension "d354" = 0.2
  dimension "d355" = 0.06
  dimension "d356" = 0.1
  dimension "d357" = 0.35
  dimension "d358" = 0.25
  dimension "d359" = 0.1
  dimension "d360" = 0.1
  dimension "d361" = 0.1
  dimension "d362" = 0.1
  dimension "d363" = 0.25
  dimension "d364" = 0.045
  dimension "d366" = 0.13
  dimension "d367" = 0.1
  dimension "d368" = 0.075
  dimension "d369" = 0.1
  dimension "d370" = 0.25
  dimension "d371" = 0.1
  dimension "d372" = 1.075
  dimension "d373" = 0.125
  dimension "d374" = 0.1
  dimension "d375" = 0.125
  dimension "d376" = 0.125
  dimension "d377" = 0.175
  dimension "d378" = 0.275
  dimension "d379" = 0.125
  dimension "d380" = 0.075
  dimension "d381" = 0.1
  dimension "d382" = 0.075
  dimension "d383" = 0.2
  constraint vertical L0
  constraint perpendicular L1 L2
  constraint coincident L4.start L8.end
  constraint coincident L9.start L16.end
  constraint tangent L20 A0
  constraint tangent L17 A0
  constraint tangent L17 A1
  constraint tangent L18 A1
  constraint tangent L18 A2
  constraint tangent L19 A2
  constraint tangent L19 A3
  constraint tangent L20 A3
  constraint tangent L23 A4
  constraint tangent L24 A4
  constraint tangent L21 A5
  constraint tangent L24 A5
  constraint tangent L22 A6
  constraint tangent L23 A6
  constraint tangent L21 A7
  constraint tangent L22 A7
  constraint parallel L0 L28
  constraint tangent L25 A8
  constraint tangent L26 A8
  constraint tangent L26 A9
  constraint tangent L27 A9
  constraint tangent L27 A10
  constraint tangent L28 A10
  constraint tangent L25 A11
  constraint tangent L29 A11
  constraint tangent L28 A12
  constraint tangent L29 A12
  constraint vertical L32
  constraint horizontal L34
  constraint parallel L34 L35
  constraint tangent L32 A13
  constraint tangent L33 A13
  constraint tangent L30 A14
  constraint tangent L35 A14
  constraint tangent L30 A15
  constraint tangent L31 A15
  constraint tangent L31 A16
  constraint tangent L32 A16
  constraint parallel L37 L38
  constraint tangent L36 A17
  constraint tangent L37 A18
  constraint coincident A17.end A18.start
  constraint tangent L36 A19
  constraint tangent L40 A19
  constraint tangent L38 A20
  constraint tangent L39 A20
  constraint equal A19 A20
  constraint tangent L39 A21
  constraint tangent L40 A21
  constraint coincident L41.start L46.end
  constraint parallel L0 L47
  constraint perpendicular L0 L48
  constraint tangent L47 A22
  constraint tangent L52 A22
  constraint tangent L51 A23
  constraint tangent L52 A23
  constraint equal A22 A23
  constraint tangent L50 A24
  constraint tangent L51 A24
  constraint tangent L49 A25
  constraint tangent L50 A25
  constraint tangent L48 A26
  constraint tangent L49 A26
  constraint tangent L47 A27
  constraint tangent L48 A27
  constraint coincident L53.start L58.end
  constraint coincident L59.start L65.end
  constraint coincident L66.start L74.end
  constraint coincident L75.start L83.end
  constraint tangent L84 A28
  constraint tangent L89 A28
  constraint tangent L84 A29
  constraint tangent L85 A29
  constraint tangent L85 A30
  constraint tangent L86 A30
  constraint tangent L86 A31
  constraint tangent L87 A31
  constraint tangent L87 A32
  constraint tangent L88 A32
  constraint tangent L88 A33
  constraint tangent L89 A33
  constraint perpendicular L91 L92
  constraint tangent L90 A34
  constraint tangent L93 A34
  constraint tangent L92 A35
  constraint tangent L93 A35
  constraint tangent L91 A36
  constraint tangent L92 A36
  constraint tangent L90 A37
  constraint tangent L91 A37
  constraint coincident L1 L94.start
  constraint coincident L3 L94.end
  constraint perpendicular L1 L94
  measures "d348" radius of A0
  measures "d349" radius of A1
  measures "d350" radius of A2
  measures "d351" radius of A3
  measures "d352" radius of A4
  measures "d353" radius of A5
  measures "d354" radius of A6
  measures "d355" radius of A7
  measures "d356" radius of A8
  measures "d357" radius of A9
  measures "d358" radius of A10
  measures "d359" radius of A11
  measures "d360" radius of A12
  measures "d361" radius of A13
  measures "d362" radius of A14
  measures "d363" radius of A15
  measures "d364" radius of A16
  measures "d366" radius of A18
  measures "d367" radius of A19
  measures "d368" radius of A21
  measures "d369" radius of A22
  measures "d370" radius of A24
  measures "d371" radius of A25
  measures "d372" radius of A26
  measures "d373" radius of A27
  measures "d374" radius of A28
  measures "d375" radius of A29
  measures "d376" radius of A30
  measures "d377" radius of A31
  measures "d378" radius of A32
  measures "d379" radius of A33
  measures "d380" radius of A34
  measures "d381" radius of A35
  measures "d382" radius of A36
  measures "d383" radius of A37
ref_plane "WorkPlane4" through (-59.2873, 0, 21.1488) normal (0, -1, 0) x (1, 0, 0)